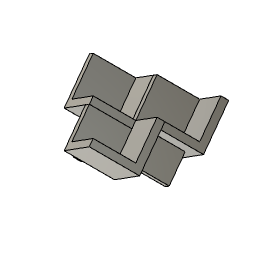
model (Autodesk Fusion 360 design; units mm, degrees)
Autodesk Fusion 360 part; units mm, degrees
sketch "leaf" plane through (0, 0, 0) normal (0, 0, 1) x (1, 0, 0) in component "base"
  line L0 (146.626, 146.626) -> (446.626, 146.626)
  line L1 (446.626, 146.626) -> (446.626, 446.626)
  line L2 (446.626, 446.626) -> (146.626, 446.626)
  line L3 (146.626, 446.626) -> (146.626, 146.626)
  line L4 (192.6635, 446.626) -> (192.6635, 192.6635)
  line L5 (192.6635, 192.6635) -> (446.626, 192.6635)
  line L6 (192.6635, 319.6448) -> (146.626, 319.6448) construction
  line L7 (319.6448, 192.6635) -> (319.6448, 146.626) construction
  line L8 (0, 0) -> (146.626, 146.626) construction
  line L9 (146.626, 146.626) -> (192.6635, 192.6635) construction
  dimension "d3" = 46.0375
  dimension "d4" = 300
  dimension "d5" = 207.3605
  constraint horizontal L0
  constraint vertical L1
  constraint horizontal L2
  constraint vertical L3
  constraint coincident L2 L4.start
  constraint perpendicular L2 L4
  constraint coincident L1 L5.end
  constraint perpendicular L1 L5
  constraint equal L1 L2
  constraint midpoint L4 L6.start
  constraint coincident L3 L6.end
  constraint perpendicular L3 L6
  constraint midpoint L5 L7.start
  constraint coincident L0 L7.end
  constraint perpendicular L0 L7
  constraint equal L6 L7
  constraint coincident L8.start origin
  constraint collinear L8 L9
  measures "d3" distance of L3 L4
  measures "d4" distance of L1.end L2.end
  measures "d5" distance of L0.start L8.start
extrude "Extrude1" add sketch "leaf" along normal blind 300 contours L0 L1 L2 L3 L4 L5 makes body 1 in component "base"
extrude "Extrude2" add sketch "leaf" along normal blind 46.0375 contours L1 L2 L4 L5 bodies 1 in component "base"
ref_plane "WorkPlane1" through (146.626, 146.626, 0) normal (-0.707107, 0.707107, 0) x (-0.707107, -0.707107, 0) in component "base"
sketch "axis" plane through (0, 0, 0) normal (0, 0, 1) x (1, 0, 0) in component "base"
  line L0 (0, 0) -> (146.626, 146.626)
  line L1 (146.626, 146.626) -> (264.8025, 28.4495) construction
  point P0 (146.626, 146.626)
  constraint coincident P0 L0.end
  constraint perpendicular L0 L1
sketch "leaf mods" plane through (0, 146.626, 0) normal (0, -1, 0) x (1, 0, 0) in component "base"
  line L0 (146.626, 0) -> (446.626, 0)
  line L1 (446.626, 0) -> (446.626, 300)
  line L2 (446.626, 300) -> (146.626, 300)
  line L3 (146.626, 300) -> (146.626, 0)
  line L4 (273.6073, 253.9625) -> (319.6448, 253.9625)
  line L5 (319.6448, 253.9625) -> (319.6448, 46.0375)
  line L6 (319.6448, 46.0375) -> (273.6073, 46.0375)
  line L7 (273.6073, 46.0375) -> (273.6073, 253.9625)
  line L8 (146.626, 150) -> (273.6073, 150) construction
  line L9 (319.6448, 150) -> (446.626, 150) construction
  line L10 (146.626, 0) -> (446.626, 0) construction
  line L11 (146.626, 300) -> (446.626, 300)
  line L12 (446.626, 300) -> (446.626, 253.9625)
  line L13 (446.626, 253.9625) -> (146.626, 253.9625)
  line L14 (146.626, 253.9625) -> (146.626, 300)
  dimension "d22" = 46.0375
  constraint horizontal L4
  constraint vertical L5
  constraint horizontal L6
  constraint vertical L7
  constraint midpoint L3 L8.start
  constraint midpoint L7 L8.end
  constraint midpoint L5 L9.start
  constraint midpoint L1 L9.end
  constraint collinear L8 L9
  constraint equal L8 L9
  constraint horizontal L11
  constraint vertical L12
  constraint horizontal L13
  constraint vertical L14
  constraint coincident L1 L12.end
  constraint coincident L2.end L3.start
  constraint collinear L4 L13
  constraint equal L4 L12
  measures "d22" distance of L4.start L4.end
extrude "Extrude5" cut sketch "leaf mods" against normal up to surface (46.0375 mm away) contours L1 L2 L3 L4 L11 L12 L13 L14 bodies 1 in component "base"
extrude "Extrude4" add sketch "leaf mods" along normal blind 190 contours L4 L5 L6 L7 L13 bodies 1 in component "base"
ref_plane "WorkPlane4" through (192.6635, 192.6635, 300) normal (0, -0.707107, 0.707107) x (1, 0, 0) in component "base"
ref_plane "WorkPlane5" through (192.6635, 192.6635, 300) normal (-0.707107, 0.707107, 0) x (-0.707107, -0.707107, 0) in component "base"
draft "Draft1" angle 45 neutral plane through (0, 0, 300) pull (0, 0, 1) 1 faces at (161.9719, 192.6635, 284.6542) on bodies 1 in component "base"
sketch "Sketch7" plane through (192.6635, 192.6635, 300) normal (-0.707107, 0.707107, 0) x (-0.707107, -0.707107, 0) in component "base"
  line L0 (0, 0) -> (65.1069, 0)
  line L1 (65.1069, 0) -> (65.1069, -46.0375)
  line L2 (65.1069, -46.0375) -> (0, -46.0375)
  line L3 (0, -46.0375) -> (0, 0)
  point P0 (65.1069, -46.0375)
  constraint horizontal L0
  constraint vertical L1
  constraint horizontal L2
  constraint vertical L3
  constraint coincident P0 L1.end
  constraint coincident L0.start L3.end
extrude "Extrude6" cut sketch "Sketch7" against normal up to surface (32.5534 mm away) bodies 1 in component "base"
move_body "Move3" bodies 1 to x (0.788672, -0.211328, 0.577353) y (-0.211328, 0.788672, 0.577353) z (-0.577353, -0.577353, 0.577345) at (61.9723, 61.9723, -169.31) in component "base"
pattern_circular "C-Pattern1" count 3 over 360 about axis through (0, 0, 1.75) along (0, 0, 1) of bodies 1 makes body 2 at (-300.2937, 153.6685, 173.2059) makes body 3 at (17.066, -336.8963, 173.2059) in component "base"
component "base" placed x (1, 0, 0) y (0, 1, 0) z (0, 0, 1) at (0, 0, 0)
equation "thickness = 29 / 16 * 1\""
equation "cubeSize = 300 mm"
equation "d3 = thickness"
equation "d4 = cubeSize"
equation "d5 = sin(compoundAngle) * ( cubeSize - thickness )"
equation "d6 = cubeSize"
equation "d8 = thickness"
equation "compoundAngle = 54.736 deg"
equation "d18 = compoundAngle"
equation "d22 = thickness"
